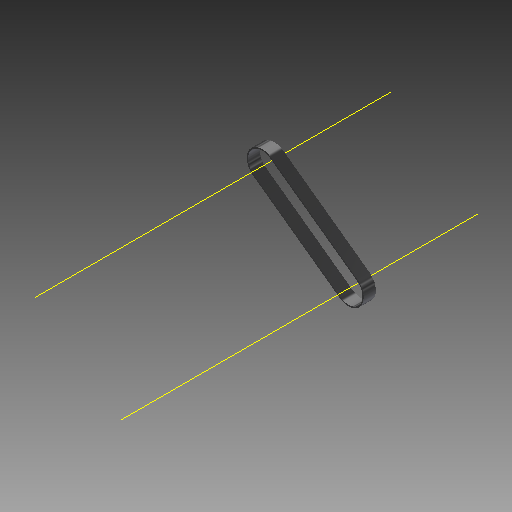
# Autodesk Inventor part: Synchronous Belt
Saved by Autodesk Inventor 2019.4 (Build 234330000, 330)
## iProperties
Created: 2020-01-27
Part Number: Synchronous Belt
Material: Rubber
Document SubType Name: Modeling
Designer: admin
Density: 1 g/cm^3
Appearance: Rubber - Black - Version 1.1
CustomPartVersion: 1
Author: admin
Autodesk Inventor part; units mm, degrees
sketch "Sketch Path" plane through (0, 0, 0) normal (0, 0, 1) x (1, 0, 0)
  arc A0 (147.128938, -61.81703) -> (161.116902, -42.471009) centre (154.12292, -52.144019) ccw
  arc A1 (90.210032, 8.797557) -> (76.222068, -10.548464) centre (83.21605, -0.875454) ccw
  line L0 (90.210032, 8.797557) -> (161.116902, -42.471009)
  line L1 (147.128938, -61.81703) -> (76.222068, -10.548464)
  constraints: 4 end point, 4 point on circle, 2 centre point
ref_plane "Cross Section Plane" through (161.116902, -42.471009, 0) normal (-0.8103642, 0.5859265, 0) x (0, 0, 1)
ref_plane "Work Plane2" through (154.12292, -52.144019, 0) normal (-1, 0, 0) x (0, 0, 1)
ref_plane "Work Plane3" through (83.21605, -0.875454, 0) normal (0.6691306, -0.7431448, 0) x (0, 0, 1)
sketch "Cross Section" plane through (161.116902, -42.471009, 0) normal (-0.8103642, 0.5859265, 0) x (0, 0, 1)
  line L0 (-5, 0.5) -> (5, 0.5)
  line L1 (5, 0.5) -> (5, -0.5)
  line L2 (5, -0.5) -> (-5, -0.5)
  line L3 (-5, -0.5) -> (-5, 0.5)
  line L4 (-5, 0) -> (5, 0) construction
  point P0 (0, 0)
  point P1 (0, 0)
  dimension "d0" = 10
  dimension "d4" = 0.5
  dimension "d5" = 0.5
  constraints: 10 end point, 3 midpoint, 2 parallel, 1 coincident, 1 horizontal, 1 perpendicular, 1 other
  measures "d0" distance between parallel lines of L1 L3
  measures "d4" distance between parallel lines of L2 L4
  measures "d5" distance between parallel lines of L4 L0
sweep "Belt" add profiles "Cross Section" path "Sketch Path" path curves L1 A1 L0 A0
equation "\"d0\" = da_B"
equation "\"d4\" = da_a"
equation "\"d5\" = da_a2"
equation "\"da_B\" = 10"
equation "\"da_pb\" = 5"
equation "\"da_a\" = 0.5"
equation "\"da_S\" = 2.65"
equation "\"da_Beta\" = 20deg"
equation "\"da_Ht\" = 1.2"
equation "\"da_H\" = 2.2"
equation "\"da_a2\" = 0.5"
body "Solid1"
